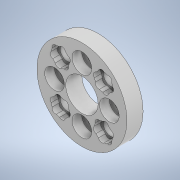
# Autodesk Inventor part: Inner_support_stand
Saved by Autodesk Inventor 2020.4 (Build 244396000, 396)
## iProperties
Created: 2021-09-25
Part Number: Inner_support_stand
Material: アルミニウム 2014-T4
Document SubType Name: Modeling
Designer: Masato
Density: 2.8 g/cm^3
Appearance: 滑らか - 淡い灰色
Author: Masato
Autodesk Inventor part; units mm, degrees
ref_plane "YZ Plane" through (0, 0, 0) normal (1, 0, 0) x (0, 1, 0)
ref_plane "XZ Plane" through (0, 0, 0) normal (0, 1, 0) x (-1, 0, 0)
ref_plane "XY Plane" through (0, 0, 0) normal (0, 0, 1) x (1, 0, 0)
derived "Inner_flange.ipt"
sketch "スケッチ1" plane through (0, 0, 0) normal (0, 0, 1) x (1, 0, 0)
  circle A0 centre (0, 0) radius 13.95
  line L0 (0, 13.95) -> (0, -13.95) construction
  circle A1 centre (0, 8.5) radius 1.35
  circle A2 centre (-8.5, 0) radius 1.35
  circle A3 centre (0, -8.5) radius 1.35
  circle A4 centre (8.5, 0) radius 1.35
  circle A5 centre (0, 0) radius 5 construction
  circle A6 centre (0, 0) radius 5.01
  circle A7 centre (-6.6998, 6.6998) radius 2.25
  line L1 (-9.8641, 9.8641) -> (9.8641, -9.8641) construction
  line L2 (-8.9534, 8.9534) -> (-5.875, 9.7782)
  line L3 (-5.875, 9.7782) -> (-3.6215, 7.5247)
  line L4 (-3.6215, 7.5247) -> (-4.4463, 4.4463)
  line L5 (-4.4463, 4.4463) -> (-7.5247, 3.6215)
  line L6 (-7.5247, 3.6215) -> (-9.7782, 5.875)
  line L7 (-9.7782, 5.875) -> (-8.9534, 8.9534)
  arc A8 (-7.9391, 9.2251) -> (-9.2251, 7.9391) centre (-8.2109, 8.2109) ccw
  arc A9 (-9.5065, 6.8892) -> (-9.0358, 5.1325) centre (-8.764, 6.1467) ccw
  arc A10 (-8.2671, 4.3639) -> (-6.5105, 3.8932) centre (-7.2529, 4.6357) ccw
  arc A11 (-5.4605, 4.1745) -> (-4.1745, 5.4605) centre (-5.1888, 5.1888) ccw
  arc A12 (-3.8932, 6.5105) -> (-4.3639, 8.2671) centre (-4.6357, 7.2529) ccw
  arc A13 (-5.1325, 9.0358) -> (-6.8892, 9.5065) centre (-6.1467, 8.764) ccw
  line L8 (-9.8641, -9.8641) -> (9.8641, 9.8641) construction
  circle A14 centre (-6.6998, -6.6998) radius 2.25
  arc A15 (-4.1745, -5.4605) -> (-5.4605, -4.1745) centre (-5.1888, -5.1888) ccw
  line L9 (-4.4463, -4.4463) -> (-3.6215, -7.5247)
  line L10 (-7.5247, -3.6215) -> (-4.4463, -4.4463)
  arc A16 (-4.3639, -8.2671) -> (-3.8932, -6.5105) centre (-4.6357, -7.2529) ccw
  line L11 (-3.6215, -7.5247) -> (-5.875, -9.7782)
  arc A17 (-6.8892, -9.5065) -> (-5.1325, -9.0358) centre (-6.1467, -8.764) ccw
  line L12 (-8.9534, -8.9534) -> (-9.7782, -5.875)
  line L13 (-5.875, -9.7782) -> (-8.9534, -8.9534)
  arc A18 (-9.2251, -7.9391) -> (-7.9391, -9.2251) centre (-8.2109, -8.2109) ccw
  arc A19 (-9.0358, -5.1325) -> (-9.5065, -6.8892) centre (-8.764, -6.1467) ccw
  arc A20 (-6.5105, -3.8932) -> (-8.2671, -4.3639) centre (-7.2529, -4.6357) ccw
  line L14 (-9.7782, -5.875) -> (-7.5247, -3.6215)
  line L15 (9.8641, -9.8641) -> (-9.8641, 9.8641) construction
  circle A21 centre (6.6998, -6.6998) radius 2.25
  arc A22 (5.4605, -4.1745) -> (4.1745, -5.4605) centre (5.1888, -5.1888) ccw
  line L16 (4.4463, -4.4463) -> (7.5247, -3.6215)
  line L17 (3.6215, -7.5247) -> (4.4463, -4.4463)
  arc A23 (8.2671, -4.3639) -> (6.5105, -3.8932) centre (7.2529, -4.6357) ccw
  line L18 (7.5247, -3.6215) -> (9.7782, -5.875)
  arc A24 (9.5065, -6.8892) -> (9.0358, -5.1325) centre (8.764, -6.1467) ccw
  line L19 (8.9534, -8.9534) -> (5.875, -9.7782)
  line L20 (9.7782, -5.875) -> (8.9534, -8.9534)
  arc A25 (7.9391, -9.2251) -> (9.2251, -7.9391) centre (8.2109, -8.2109) ccw
  arc A26 (5.1325, -9.0358) -> (6.8892, -9.5065) centre (6.1467, -8.764) ccw
  arc A27 (3.8932, -6.5105) -> (4.3639, -8.2671) centre (4.6357, -7.2529) ccw
  line L21 (5.875, -9.7782) -> (3.6215, -7.5247)
  line L22 (9.8641, 9.8641) -> (-9.8641, -9.8641) construction
  circle A28 centre (6.6998, 6.6998) radius 2.25
  arc A29 (4.1745, 5.4605) -> (5.4605, 4.1745) centre (5.1888, 5.1888) ccw
  line L23 (4.4463, 4.4463) -> (3.6215, 7.5247)
  line L24 (7.5247, 3.6215) -> (4.4463, 4.4463)
  arc A30 (4.3639, 8.2671) -> (3.8932, 6.5105) centre (4.6357, 7.2529) ccw
  line L25 (3.6215, 7.5247) -> (5.875, 9.7782)
  arc A31 (6.8892, 9.5065) -> (5.1325, 9.0358) centre (6.1467, 8.764) ccw
  line L26 (8.9534, 8.9534) -> (9.7782, 5.875)
  line L27 (5.875, 9.7782) -> (8.9534, 8.9534)
  arc A32 (9.2251, 7.9391) -> (7.9391, 9.2251) centre (8.2109, 8.2109) ccw
  arc A33 (9.0358, 5.1325) -> (9.5065, 6.8892) centre (8.764, 6.1467) ccw
  arc A34 (6.5105, 3.8932) -> (8.2671, 4.3639) centre (7.2529, 4.6357) ccw
  line L28 (9.7782, 5.875) -> (7.5247, 3.6215)
  circle A35 centre (0, 8.5) radius 3.05
  circle A36 centre (-8.5, 0) radius 3.05
  circle A37 centre (0, -8.5) radius 3.05
  circle A38 centre (8.5, 0) radius 3.05
  point P0 (-9.7782, 5.875)
  point P1 (-7.5247, 3.6215)
  point P2 (-4.4463, 4.4463)
  point P3 (-3.6215, 7.5247)
  point P4 (-5.875, 9.7782)
  point P5 (-4.4463, -4.4463)
  point P6 (-3.6215, -7.5247)
  point P7 (-5.875, -9.7782)
  point P8 (-9.7782, -5.875)
  point P9 (-7.5247, -3.6215)
  point P10 (4.4463, -4.4463)
  point P11 (7.5247, -3.6215)
  point P12 (9.7782, -5.875)
  point P13 (5.875, -9.7782)
  point P14 (3.6215, -7.5247)
  point P15 (4.4463, 4.4463)
  point P16 (3.6215, 7.5247)
  point P17 (5.875, 9.7782)
  point P18 (9.7782, 5.875)
  point P19 (7.5247, 3.6215)
  point P20 (-5.1325, 9.0358)
  point P21 (-4.3639, 8.2671)
  point P22 (-3.8932, 6.5105)
  point P23 (-4.1745, 5.4605)
  point P24 (-6.5105, 3.8932)
  point P25 (-9.0358, 5.1325)
  point P26 (-6.8892, 9.5065)
  point P27 (-9.0358, -5.1325)
  point P28 (-8.2671, -4.3639)
  point P29 (-6.5105, -3.8932)
  point P30 (-5.4605, -4.1745)
  point P31 (-4.1745, -5.4605)
  point P32 (-3.8932, -6.5105)
  point P33 (-4.3639, -8.2671)
  point P34 (-5.1325, -9.0358)
  point P35 (-9.5065, -6.8892)
  point P36 (5.1325, -9.0358)
  point P37 (4.3639, -8.2671)
  point P38 (3.8932, -6.5105)
  point P39 (4.1745, -5.4605)
  point P40 (5.4605, -4.1745)
  point P41 (6.5105, -3.8932)
  point P42 (9.0358, -5.1325)
  point P43 (6.8892, -9.5065)
  point P44 (9.0358, 5.1325)
  point P45 (6.5105, 3.8932)
  point P46 (5.4605, 4.1745)
  point P47 (3.8932, 6.5105)
  point P48 (4.3639, 8.2671)
  point P49 (5.1325, 9.0358)
  point P50 (9.5065, 6.8892)
  dimension "d3" = 4.5
  dimension "d4" = 45
  dimension "d5" = 8.95
  dimension "d6" = 10
  dimension "d7" = 9.475
  dimension "d8" = 5.52
  dimension "d9" = 1.05
  dimension "d12" = 360
  dimension "d16" = 360
  dimension "d20" = 6.1
  dimension "d21" = 6.1
  dimension "d22" = 6.1
  dimension "d23" = 6.1
  measures "d3" diameter of A7
  measures "d4" angle of L1 L0
  measures "d5" radial gap between concentric circles of A5 A0
  measures "d6" diameter of A5
  measures "d7" distance of point (0, 0) A7.centre
  measures "d8" distance between parallel lines of L6 L3
  measures "d9" radius of A8
  measures "d20" diameter of A35
  measures "d21" diameter of A36
  measures "d22" diameter of A37
  measures "d23" diameter of A38
extrude "押し出し1" add sketch "スケッチ1" along normal blind 5 contours A0
extrude "押し出し2" add sketch "スケッチ1" along normal blind 2.8 contours A8 L2 | L2 L3 L4 L5 L6 L7 | L7 A8 | A13 L2 | L7 A9 | A13 L3 | L6 A9 | A12 L3 | L6 A10 | A12 L4 | L5 A10 | A11 L4 | L5 A11 | L9 A15 | L9 L11 L13 L12 L14 L10 | L10 A15 | A16 L9 | A16 L11 | L10 A20 | L14 A20 | A17 L11 | A17 L13 | L14 A19 | L12 A19 | A18 L13 | A18 L12 | L16 A22 | L16 L18 L20 L19 L21 L17 | L17 A22 | A23 L16 | A23 L18 | L17 A27 | L21 A27 | A24 L18 | A24 L20 | L21 A26 | L19 A26 | A25 L20 | A25 L19 | L23 A29 | L23 L25 L27 L26 L28 L24 | L24 A29 | A30 L23 | A30 L25 | L24 A34 | L28 A34 | A31 L25 | A31 L27 | L28 A33 | L26 A33 | A32 L27 | A32 L26
extrude "押し出し3" add sketch "スケッチ1" along normal blind 2 contours A35 | A36 | A37 | A38
equation "\"d7\" = 0.5 * d6 + 0.5 * d5"
equation "\"d21\" = d20"
equation "\"d22\" = d20"
equation "\"d23\" = d20"
